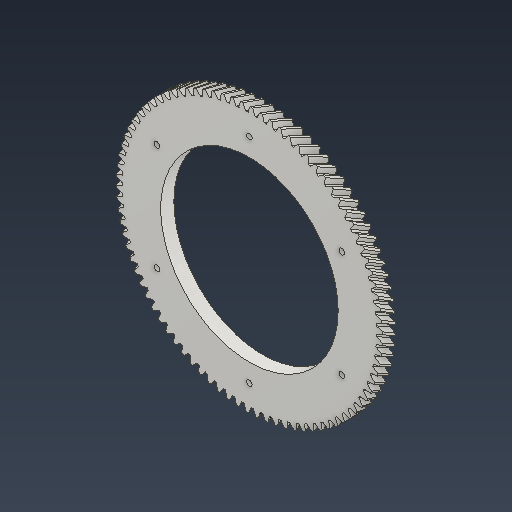
# Autodesk Inventor part: Цилиндрическое зубчатое зацепление2
Saved by Autodesk Inventor 2026 (Build 300175000, 175)
## iProperties
CustomPartVersion: 1
Created: 2025-11-26
Part Number: Цилиндрическое зубчатое зацепление2
Material: Steel
Document SubType Name: Modeling
Designer: Phantom
Categories: <?xml version="1.0" encoding="UTF-16"?> <MemberInstance><Categories><FamilyTemplate><FamilyTemplateParameter ValueType="xs:double" Id="1" ObjectReferenceKey="da_z" ObjectType="kUserParameterObject"/><FamilyTemplateParameter ValueType="xs:double" Id="2" ObjectReferenceKey="da_b" ObjectType="kUserParameterObject"/><FamilyTemplateParameter ValueType="xs:double" Id="3" ObjectReferenceKey="da_beta" ObjectType="kUserParameterObject"/><FamilyTemplateParameter ValueType="xs:double" Id="4" ObjectReferenceKey="da_da" ObjectType="kUserParameterObject"/><FamilyTemplateParameter ValueType="xs:double" Id="5" ObjectReferenceKey="da_aw" ObjectType="kUserParameterObject"/><FamilyTemplateParameter ValueType="xs:string" Id="6" ObjectReferenceKey="EAIAABAAAACIAQAAAAAAAIAAAAAAAAAA" ObjectType="83910656" SubObjectId="SurfaceGeometry"/></FamilyTemplate><ParamToTemplateMap><ParamToTemplate CategoryParameter="//CategoryParameter[@InternalName='046C89C9-8512-4d59-83FE-43B91F4F132A']" TemplateParameter="1"/><ParamToTemplate CategoryParameter="//CategoryParameter[@InternalName='2552DF32-E462-4b46-AEBF-C6C7768E72AC']" TemplateParameter="2"/><ParamToTemplate CategoryParameter="//CategoryParameter[@InternalName='C9EE641D-15FC-4fae-A226-E94C4372FDD7']" TemplateParameter="3"/><ParamToTemplate><ParamToTemplate CategoryParameter="//CategoryParameter[@InternalName='00B6519A-459B-49c7-AD84-2E56D39A5744']" ConstantValue="-0.044335"/></ParamToTemplate><ParamToTemplate><ParamToTemplate CategoryParameter="//CategoryParameter[@InternalName='04B31F0E-C7A6-4894-AA32-9629BEFACF47']" ConstantValue="1.000000"/></ParamToTemplate><ParamToTemplate><ParamToTemplate CategoryParameter="//CategoryParameter[@InternalName='43CBEC2E-7847-49e7-A936-2F7889FCB2D9']" ConstantValue="0.250000"/></ParamToTemplate><ParamToTemplate><ParamToTemplate CategoryParameter="//CategoryParameter[@InternalName='B1EFC894-105D-4ebd-86BF-FA20ED196853']" ConstantValue="0.350000"/></ParamToTemplate><ParamToTemplate><ParamToTemplate CategoryParameter="//CategoryParameter[@InternalName='51175063-3D10-4879-93E8-6246FE8B403D']" ConstantValue="2060000000.000000"/></ParamToTemplate><ParamToTemplate><ParamToTemplate CategoryParameter="//CategoryParameter[@InternalName='A3A52E27-4454-46a9-B0BD-C932399B70AF']" ConstantValue="0.300000"/></ParamToTemplate><ParamToTemplate><ParamToTemplate CategoryParameter="//CategoryParameter[@InternalName='91B76062-C214-41d9-B1B9-14D2AB99603D']" ConstantValue="0.200000"/></ParamToTemplate><ParamToTemplate><ParamToTemplate CategoryParameter="//CategoryParameter[@InternalName='374E806E-8B8A-4dda-A9AA-1039D6500AD2']" ConstantValue="5.000000"/></ParamToTemplate><ParamToTemplate><ParamToTemplate CategoryParameter="//CategoryParameter[@InternalName='2D373A89-B862-43d6-8D0B-0CBF12AB9F6C']" ConstantValue="0.349066"/></ParamToTemplate><ParamToTemplate CategoryParameter="//CategoryParameter[@InternalName='37777632-D6A2-4fac-9D53-DB8ACD95C989']" TemplateParameter="4"/><ParamToTemplate CategoryParameter="//CategoryParameter[@InternalName='FD1017F1-B727-4f7e-9707-0F86F1FF9423']" TemplateParameter="5"/><ParamToTemplate><ParamToTemplate CategoryParameter="//CategoryParameter[@InternalName='9E1B4470-B2D3-4ff1-B813-535BB4CDF51A']" ConstantValue="3520000.000000"/></ParamToTemplate><ParamToTemplate><ParamToTemplate CategoryParameter="//CategoryParameter[@InternalName='F8452263-BFF6-458c-9FB1-07C4B99E95CD']" ConstantValue="11400000.000000"/></ParamToTemplate><ParamToTemplate><ParamToTemplate CategoryParameter="//CategoryParameter[@InternalName='3E3BB259-FD49-497f-8171-6EBC954A3479']" ConstantValue="2.000000"/></ParamToTemplate><ParamToTemplate CategoryParameter="//CategoryParameter[@InternalName='27C3BAF2-7550-4e4b-AE2C-0DB134B7D9B7']" TemplateParameter="6"/></ParamToTemplateMap><Category DisplayName="Gear" InternalName="DC85795E-93AB-48d5-8EEE-5A27447B64BD" Mnemonic="Gear"><CategoryParameter DisplayName="z" InternalName="046C89C9-8512-4d59-83FE-43B91F4F132A" Mnemonic="z"/><CategoryParameter DisplayName="b" InternalName="2552DF32-E462-4b46-AEBF-C6C7768E72AC" Mnemonic="b"/><CategoryParameter DisplayName="||b|" InternalName="C9EE641D-15FC-4fae-A226-E94C4372FDD7" Mnemonic="beta"/><CategoryParameter DisplayName="x" InternalName="00B6519A-459B-49c7-AD84-2E56D39A5744" Mnemonic="x"/><CategoryParameter DisplayName="a*" InternalName="04B31F0E-C7A6-4894-AA32-9629BEFACF47" Mnemonic="a"/><CategoryParameter DisplayName="c*" InternalName="43CBEC2E-7847-49e7-A936-2F7889FCB2D9" Mnemonic="c"/><CategoryParameter DisplayName="r|.f|*" InternalName="B1EFC894-105D-4ebd-86BF-FA20ED196853" Mnemonic="rf"/><CategoryParameter DisplayName="E" InternalName="51175063-3D10-4879-93E8-6246FE8B403D" Mnemonic="E"/><CategoryParameter DisplayName="||m|" InternalName="A3A52E27-4454-46a9-B0BD-C932399B70AF" Mnemonic="mi"/><Category DisplayName="SpurGear" InternalName="26C5A22E-A91E-4dfd-A3B3-23CCAFAE1764" Mnemonic="SpurGear"><CategoryParameter DisplayName="m" InternalName="91B76062-C214-41d9-B1B9-14D2AB99603D" Mnemonic="m"/><CategoryParameter DisplayName="P" InternalName="374E806E-8B8A-4dda-A9AA-1039D6500AD2" Mnemonic="PP"/><CategoryParameter DisplayName="||a|" InternalName="2D373A89-B862-43d6-8D0B-0CBF12AB9F6C" Mnemonic="alpha"/><CategoryParameter DisplayName="d|.a|" InternalName="37777632-D6A2-4fac-9D53-DB8ACD95C989" Mnemonic="da"/><CategoryParameter DisplayName="a|.w|" InternalName="FD1017F1-B727-4f7e-9707-0F86F1FF9423" Mnemonic="aw"/><CategoryParameter DisplayName="||s||.Flim|" InternalName="9E1B4470-B2D3-4ff1-B813-535BB4CDF51A" Mnemonic="sFlim"/><CategoryParameter DisplayName="||s||.Hlim|" InternalName="F8452263-BFF6-458c-9FB1-07C4B99E95CD" Mnemonic="sHlim"/><CategoryParameter DisplayName="тип" InternalName="3E3BB259-FD49-497f-8171-6EBC954A3479" Mnemonic="type"/><CategoryParameter DisplayName="PitchDiameter" InternalName="27C3BAF2-7550-4e4b-AE2C-0DB134B7D9B7" Mnemonic="IDS_PITCHDIAM"/></Category></Category></Categories></MemberInstance>
Density: 1 g/cm^3
Appearance: Steel
d16: 120,000 мм
d17: 0,000 мм
d41: 0,000 мм
d43: 120,000 мм
d46: 120,000 мм
d47: 0,000 мм
d48: 0,000 мм
Author: Phantom
Autodesk Inventor part; units mm, degrees
(part 1 of 2)
sketch "Sketch1" plane through (0, 0, 0) normal (0, 0, 1) x (1, 0, 0)
  circle A0 centre (0, 0) radius 101.2154
  dimension "d0" = 202.4308
  constraints: 1 centre point
  measures "d0" diameter of A0
extrude "Extrusion1" add sketch "Sketch1" along normal blind 10
ref_plane "Work Plane2" through (0, 0, 5) normal (0, 0, 1) x (-0.9983104, -0.0581068, 0)
sketch "Sketch2" plane through (0, 0, 0) normal (0, 0, -1) x (-1, 0, 0)
  circle A0 centre (0, 0) radius 101.2154 projected
  circle A1 centre (0, 0) radius 99.3042
  dimension "d3" = 198.6085
  constraints: 1 centre point, 1 coincident
  measures "d3" diameter of A1
surface extrude "Средний диаметр" sketch "Sketch2" against normal through all shown no curves A1
ref_plane "Work Plane8" through (0, 0, 0) normal (0.9993328, 0.036522, 0) x (0, 0, 1)
ref_plane "Work Plane9" through (0, 0, 0) normal (1, 0, 0) x (0, 1, 0)
spur gear teeth "Цилиндрическое зубчатое зацепление" teeth 86 pitch diameter 198.6085 tip diameter 202.4308 root diameter 193.4312 face width 10 helix angle 30 hand right start plane through (0, 0, 0) normal (0, 0, -1) x (-1, 0, 0)
sketch "Эскиз3" plane through (0, 0, 10) normal (0, 0, 1) x (1, 0, 0)
  circle A0 centre (0, 0) radius 67.5
  dimension "d49" = 135
  constraints: 1 centre point, 1 coincident
  measures "d49" diameter of A0
extrude "Выдавливание2" cut sketch "Эскиз3" against normal through all
sketch "Эскиз4" plane through (0, 0, 10) normal (0, 0, 1) x (1, 0, 0)
  circle A0 centre (0, 0) radius 67.5
  arc A1 (-12.5637, 100.4326) -> (-14.3959, 100.1864) centre (0, 0) ccw
  spline S0 degree 3 poles (-8.4922, 96.342) (-8.7855, 96.3162) (-9.0787, 96.289) (-9.6648, 96.2319) (-9.9577, 96.2021) (-10.2504, 96.1708) knots 0 0 0 0 0.5 0.5 1 1 1 1
  spline S1 degree 3 poles (-1.4371, 96.7049) (-1.7315, 96.7005) (-2.0258, 96.6948) (-2.6145, 96.6807) (-2.9088, 96.6723) (-3.2031, 96.6625) knots 0 0 0 0 0.5 0.5 1 1 1 1
  spline S2 degree 3 poles (0.3447, 101.2148) (-0.0226, 100.4934) (-0.3555, 99.755) (-0.9504, 98.2491) (-1.2121, 97.4826) (-1.4371, 96.7049) knots 0 0 0 0 0.5 0.5 1 1 1 1
  arc A2 (2.1933, 101.1916) -> (0.3447, 101.2148) centre (0, 0) ccw
  spline S3 degree 3 poles (3.8614, 96.6385) (3.656, 97.4215) (3.4136, 98.1944) (2.8566, 99.7147) (2.5423, 100.4612) (2.1933, 101.1916) knots 0 0 0 0 0.5 0.5 1 1 1 1
  spline S4 degree 3 poles (5.6258, 96.5518) (5.3318, 96.5689) (5.0378, 96.5847) (4.4497, 96.6136) (4.1556, 96.6267) (3.8614, 96.6385) knots 0 0 0 0 0.5 0.5 1 1 1 1
  spline S5 degree 3 poles (7.732, 100.9196) (7.313, 100.2269) (6.9271, 99.5148) (6.2238, 98.0564) (5.9069, 97.311) (5.6258, 96.5518) knots 0 0 0 0 0.5 0.5 1 1 1 1
  arc A3 (9.5739, 100.7616) -> (7.732, 100.9196) centre (0, 0) ccw
  spline S6 degree 3 poles (10.9053, 96.0988) (10.7575, 96.8947) (10.5722, 97.6833) (10.1277, 99.2401) (9.8687, 100.0076) (9.5739, 100.7616) knots 0 0 0 0 0.5 0.5 1 1 1 1
  spline S7 degree 3 poles (12.6586, 95.8836) (12.3667, 95.9221) (12.0746, 95.9593) (11.4902, 96.0311) (11.1978, 96.0656) (10.9053, 96.0988) knots 0 0 0 0 0.5 0.5 1 1 1 1
  spline S8 degree 3 poles (15.078, 100.086) (14.6096, 99.4257) (14.1727, 98.7437) (13.3649, 97.3405) (12.9944, 96.6202) (12.6586, 95.8836) knots 0 0 0 0 0.5 0.5 1 1 1 1
  arc A4 (16.9035, 99.7939) -> (15.078, 100.086) centre (0, 0) ccw
  spline S9 degree 3 poles (17.8909, 95.0464) (17.8017, 95.851) (17.6745, 96.651) (17.3448, 98.2361) (17.1425, 99.0205) (16.9035, 99.7939) knots 0 0 0 0 0.5 0.5 1 1 1 1
  spline S10 degree 3 poles (19.6239, 94.7038) (19.3356, 94.7635) (19.047, 94.8219) (18.4694, 94.9361) (18.1803, 94.9919) (17.8909, 95.0464) knots 0 0 0 0 0.5 0.5 1 1 1 1
  spline S11 degree 3 poles (22.3436, 98.7184) (21.8283, 98.0941) (21.3428, 97.4457) (20.4346, 96.1052) (20.0126, 95.4139) (19.6239, 94.7038) knots 0 0 0 0 0.5 0.5 1 1 1 1
  arc A5 (24.1429, 98.2938) -> (22.3436, 98.7184) centre (0, 0) ccw
  spline S12 degree 3 poles (24.7811, 93.4869) (24.7509, 94.2959) (24.6824, 95.103) (24.4693, 96.708) (24.3248, 97.505) (24.1429, 98.2938) knots 0 0 0 0 0.5 0.5 1 1 1 1
  spline S13 degree 3 poles (26.4845, 93.0187) (26.2013, 93.0993) (25.9178, 93.1786) (25.35, 93.3347) (25.0657, 93.4114) (24.7811, 93.4869) knots 0 0 0 0 0.5 0.5 1 1 1 1
  spline S14 degree 3 poles (29.49, 96.824) (28.9304, 96.239) (28.3989, 95.6278) (27.3954, 94.3572) (26.9239, 93.6986) (26.4845, 93.0187) knots 0 0 0 0 0.5 0.5 1 1 1 1
  arc A6 (31.2535, 96.2693) -> (29.49, 96.824) centre (0, 0) ccw
  spline S15 degree 3 poles (31.5391, 91.4286) (31.568, 92.2376) (31.5586, 93.0476) (31.4632, 94.6638) (31.3773, 95.4693) (31.2535, 96.2693) knots 0 0 0 0 0.5 0.5 1 1 1 1
  spline S16 degree 3 poles (33.2037, 90.8373) (32.9272, 90.9384) (32.6502, 91.0382) (32.0953, 91.2353) (31.8175, 91.3326) (31.5391, 91.4286) knots 0 0 0 0 0.5 0.5 1 1 1 1
  spline S17 degree 3 poles (36.479, 94.4131) (35.8783, 93.8705) (35.3035, 93.2997) (34.2099, 92.1058) (33.6917, 91.4833) (33.2037, 90.8373) knots 0 0 0 0 0.5 0.5 1 1 1 1
  arc A7 (38.1973, 93.7311) -> (36.479, 94.4131) centre (0, 0) ccw
  spline S18 degree 3 poles (38.1289, 88.8825) (38.2167, 89.6872) (38.2664, 90.4957) (38.2893, 92.1146) (38.2624, 92.9242) (38.1973, 93.7311) knots 0 0 0 0 0.5 0.5 1 1 1 1
  spline S19 degree 3 poles (39.7459, 88.1713) (39.4774, 88.2922) (39.2085, 88.412) (38.6695, 88.6491) (38.3994, 88.7664) (38.1289, 88.8825) knots 0 0 0 0 0.5 0.5 1 1 1 1
  spline S20 degree 3 poles (43.2734, 91.4984) (42.6347, 91.0011) (42.0198, 90.4738) (40.8419, 89.3629) (40.2796, 88.7799) (39.7459, 88.1713) knots 0 0 0 0 0.5 0.5 1 1 1 1
  arc A8 (44.9373, 90.6928) -> (43.2734, 91.4984) centre (0, 0) ccw
  spline S21 degree 3 poles (44.5151, 85.8621) (44.6615, 86.6583) (44.7701, 87.461) (44.9111, 89.074) (44.9434, 89.8833) (44.9373, 90.6928) knots 0 0 0 0 0.5 0.5 1 1 1 1
  spline S22 degree 3 poles (46.0759, 85.0348) (45.817, 85.175) (45.5575, 85.3141) (45.0373, 85.5899) (44.7765, 85.7266) (44.5151, 85.8621) knots 0 0 0 0 0.5 0.5 1 1 1 1
  spline S23 degree 3 poles (49.8369, 88.0956) (49.1636, 87.6462) (48.5119, 87.1652) (47.2561, 86.1432) (46.6527, 85.6028) (46.0759, 85.0348) knots 0 0 0 0 0.5 0.5 1 1 1 1
  arc A9 (51.4376, 87.1707) -> (49.8369, 88.0956) centre (0, 0) ccw
  spline S24 degree 3 poles (50.6639, 82.3837) (50.868, 83.1671) (51.0349, 83.9597) (51.2933, 85.558) (51.3845, 86.3629) (51.4376, 87.1707) knots 0 0 0 0 0.5 0.5 1 1 1 1
  spline S25 degree 3 poles (52.1601, 81.4446) (51.9122, 81.6034) (51.6635, 81.761) (51.1648, 82.0741) (50.9147, 82.2294) (50.6639, 82.3837) knots 0 0 0 0 0.5 0.5 1 1 1 1
  spline S26 degree 3 poles (56.1346, 84.2227) (55.4302, 83.8237) (54.7451, 83.3916) (53.4181, 82.464) (52.7769, 81.969) (52.1601, 81.4446) knots 0 0 0 0 0.5 0.5 1 1 1 1
  arc A10 (57.6634, 83.1834) -> (56.1346, 84.2227) centre (0, 0) ccw
  spline S27 degree 3 poles (56.5424, 78.4657) (56.8031, 79.2321) (57.0275, 80.0104) (57.4018, 81.5856) (57.5515, 82.3817) (57.6634, 83.1834) knots 0 0 0 0 0.5 0.5 1 1 1 1
  spline S28 degree 3 poles (57.9661, 77.4199) (57.7304, 77.5963) (57.4939, 77.7717) (57.0193, 78.1203) (56.7813, 78.2935) (56.5424, 78.4657) knots 0 0 0 0 0.5 0.5 1 1 1 1
  spline S29 degree 3 poles (62.1327, 79.9005) (61.401, 79.5539) (60.6862, 79.173) (59.295, 78.3447) (58.6194, 77.8979) (57.9661, 77.4199) knots 0 0 0 0 0.5 0.5 1 1 1 1
  arc A11 (63.5816, 78.7524) -> (62.1327, 79.9005) centre (0, 0) ccw
  spline S30 degree 3 poles (62.1192, 74.129) (62.4352, 74.8743) (62.7157, 75.6342) (63.204, 77.1779) (63.4115, 77.9609) (63.5816, 78.7524) knots 0 0 0 0 0.5 0.5 1 1 1 1
  spline S31 degree 3 poles (63.4627, 72.9821) (63.2405, 73.1753) (63.0175, 73.3675) (62.5696, 73.7498) (62.3448, 73.9399) (62.1192, 74.129) knots 0 0 0 0 0.5 0.5 1 1 1 1
  spline S32 degree 3 poles (67.7993, 75.1519) (67.0443, 74.8597) (66.3036, 74.5319) (64.8556, 73.8074) (64.1492, 73.4111) (63.4627, 72.9821) knots 0 0 0 0 0.5 0.5 1 1 1 1
  arc A12 (69.1606, 73.9011) -> (67.7993, 75.1519) centre (0, 0) ccw
  spline S33 degree 3 poles (67.3645, 69.3969) (67.7341, 70.1171) (68.0693, 70.8545) (68.669, 72.3584) (68.9331, 73.1242) (69.1606, 73.9011) knots 0 0 0 0 0.5 0.5 1 1 1 1
  spline S34 degree 3 poles (68.6208, 68.1549) (68.4133, 68.3638) (68.2049, 68.5718) (67.7861, 68.9857) (67.5758, 69.1918) (67.3645, 69.3969) knots 0 0 0 0 0.5 0.5 1 1 1 1
  spline S35 degree 3 poles (73.1041, 70.0024) (72.3299, 69.7661) (71.5672, 69.4933) (70.0702, 68.8764) (69.3368, 68.5327) (68.6208, 68.1549) knots 0 0 0 0 0.5 0.5 1 1 1 1
  arc A13 (74.3705, 68.6556) -> (73.1041, 70.0024) centre (0, 0) ccw
  spline S36 degree 3 poles (72.2505, 64.2944) (72.6716, 64.9858) (73.0598, 65.6967) (73.7677, 67.1529) (74.0869, 67.8973) (74.3705, 68.6556) knots 0 0 0 0 0.5 0.5 1 1 1 1
  spline S37 degree 3 poles (73.4127, 62.9641) (73.221, 63.1876) (73.0283, 63.4102) (72.6409, 63.8536) (72.4462, 64.0745) (72.2505, 64.2944) knots 0 0 0 0 0.5 0.5 1 1 1 1
  spline S38 degree 3 poles (78.019, 64.4794) (77.2295, 64.3002) (76.449, 64.0838) (74.911, 63.5778) (74.1544, 63.2886) (73.4127, 62.9641) knots 0 0 0 0 0.5 0.5 1 1 1 1
  arc A14 (79.1836, 63.0437) -> (78.019, 64.4794) centre (0, 0) ccw
  spline S39 degree 3 poles (76.7509, 58.849) (77.2214, 59.5078) (77.6604, 60.1884) (78.4727, 61.589) (78.8455, 62.3082) (79.1836, 63.0437) knots 0 0 0 0 0.5 0.5 1 1 1 1
  spline S40 degree 3 poles (77.8129, 57.4374) (77.6381, 57.6742) (77.4622, 57.9103) (77.1081, 58.3809) (76.9301, 58.6153) (76.7509, 58.849) knots 0 0 0 0 0.5 0.5 1 1 1 1
  spline S41 degree 3 poles (82.5175, 58.6124) (81.7171, 58.4913) (80.9228, 58.3324) (79.352, 57.9401) (78.5763, 57.7069) (77.8129, 57.4374) knots 0 0 0 0 0.5 0.5 1 1 1 1
  arc A15 (83.5743, 57.0955) -> (82.5175, 58.6124) centre (0, 0) ccw
  spline S42 degree 3 poles (80.8419, 53.0895) (81.3592, 53.7122) (81.8467, 54.359) (82.7591, 55.6966) (83.1833, 56.3866) (83.5743, 57.0955) knots 0 0 0 0 0.5 0.5 1 1 1 1
  spline S43 degree 3 poles (81.798, 51.6042) (81.6409, 51.8532) (81.4827, 52.1015) (81.164, 52.5966) (81.0035, 52.8434) (80.8419, 53.0895) knots 0 0 0 0 0.5 0.5 1 1 1 1
  spline S44 degree 3 poles (86.5758, 52.4326) (85.7687, 52.3703) (84.9649, 52.2698) (83.3697, 51.9932) (82.579, 51.8172) (81.798, 51.6042) knots 0 0 0 0 0.5 0.5 1 1 1 1
  arc A16 (87.519, 50.8427) -> (86.5758, 52.4326) centre (0, 0) ccw
  spline S45 degree 3 poles (84.5015, 47.0468) (85.0629, 47.6301) (85.5964, 48.2396) (86.6039, 49.507) (87.0774, 50.1642) (87.519, 50.8427) knots 0 0 0 0 0.5 0.5 1 1 1 1
  spline S46 degree 3 poles (85.3467, 45.4956) (85.2082, 45.7554) (85.0685, 46.0146) (84.7867, 46.5317) (84.6447, 46.7896) (84.5015, 47.0468) knots 0 0 0 0 0.5 0.5 1 1 1 1
  spline S47 degree 3 poles (90.1722, 45.9731) (89.3627, 45.9699) (88.5537, 45.9283) (86.9425, 45.7689) (86.1411, 45.6511) (85.3467, 45.4956) knots 0 0 0 0 0.5 0.5 1 1 1 1
  arc A17 (90.9968, 44.3185) -> (90.1722, 45.9731) centre (0, 0) ccw
  spline S48 degree 3 poles (87.7103, 40.7531) (88.3127, 41.2938) (88.8893, 41.8628) (89.9866, 43.0532) (90.5068, 43.6741) (90.9968, 44.3185) knots 0 0 0 0 0.5 0.5 1 1 1 1
  spline S49 degree 3 poles (88.4399, 39.1443) (88.3208, 39.4136) (88.2004, 39.6823) (87.9572, 40.2185) (87.8343, 40.4861) (87.7103, 40.7531) knots 0 0 0 0 0.5 0.5 1 1 1 1
  spline S50 degree 3 poles (93.2875, 39.2683) (92.4799, 39.3242) (91.6701, 39.3418) (90.0515, 39.3004) (89.2436, 39.2414) (88.4399, 39.1443) knots 0 0 0 0 0.5 0.5 1 1 1 1
  arc A18 (93.9891, 37.558) -> (93.2875, 39.2683) centre (0, 0) ccw
  spline S51 degree 3 poles (90.4511, 34.2419) (91.0914, 34.7372) (91.7079, 35.2626) (92.8893, 36.3698) (93.4534, 36.951) (93.9891, 37.558) knots 0 0 0 0 0.5 0.5 1 1 1 1
  spline S52 degree 3 poles (91.0614, 32.5842) (90.9622, 32.8614) (90.8617, 33.1382) (90.6583, 33.6908) (90.5553, 33.9666) (90.4511, 34.2419) knots 0 0 0 0 0.5 0.5 1 1 1 1
  spline S53 degree 3 poles (95.905, 32.354) (95.1036, 32.4687) (94.2973, 32.5454) (92.68, 32.6222) (91.87, 32.6224) (91.0614, 32.5842) knots 0 0 0 0 0.5 0.5 1 1 1 1
  arc A19 (96.4799, 30.597) -> (95.905, 32.354) centre (0, 0) ccw
  spline S54 degree 3 poles (92.7093, 27.5481) (93.384, 27.9953) (94.0373, 28.4743) (95.2963, 29.4923) (95.9013, 30.0308) (96.4799, 30.597) knots 0 0 0 0 0.5 0.5 1 1 1 1
  spline S55 degree 3 poles (93.1969, 25.8502) (93.1182, 26.1339) (93.0383, 26.4173) (92.8757, 26.9833) (92.7931, 27.2659) (92.7093, 27.5481) knots 0 0 0 0 0.5 0.5 1 1 1 1
  spline S56 degree 3 poles (98.0109, 25.2671) (97.22, 25.44) (96.4214, 25.5753) (94.814, 25.77) (94.0062, 25.8293) (93.1969, 25.8502) knots 0 0 0 0 0.5 0.5 1 1 1 1
  arc A20 (98.456, 23.4728) -> (98.0109, 25.2671) centre (0, 0) ccw
  spline S57 degree 3 poles (94.4728, 20.7072) (95.1784, 21.104) (95.8649, 21.534) (97.1949, 22.4574) (97.8376, 22.9503) (98.456, 23.4728) knots 0 0 0 0 0.5 0.5 1 1 1 1
  spline S58 degree 3 poles (94.8353, 18.9783) (94.7775, 19.267) (94.7184, 19.5555) (94.5976, 20.1318) (94.5359, 20.4197) (94.4728, 20.7072) knots 0 0 0 0 0.5 0.5 1 1 1 1
  spline S59 degree 3 poles (99.5938, 18.0454) (98.8176, 18.2755) (98.031, 18.4687) (96.4422, 18.7803) (95.6408, 18.8983) (94.8353, 18.9783) knots 0 0 0 0 0.5 0.5 1 1 1 1
  arc A21 (99.9067, 16.2234) -> (99.5938, 18.0454) centre (0, 0) ccw
  spline S60 degree 3 poles (95.7323, 13.7559) (96.465, 14.1002) (97.181, 14.4789) (98.5749, 15.3027) (99.2519, 15.7474) (99.9067, 16.2234) knots 0 0 0 0 0.5 0.5 1 1 1 1
  spline S61 degree 3 poles (95.9676, 12.0052) (95.931, 12.2973) (95.8932, 12.5893) (95.8147, 13.1729) (95.7742, 13.4645) (95.7323, 13.7559) knots 0 0 0 0 0.5 0.5 1 1 1 1
  spline S62 degree 3 poles (100.6453, 10.7273) (99.888, 11.0135) (99.1176, 11.2637) (97.5558, 11.6903) (96.7652, 11.8666) (95.9676, 12.0052) knots 0 0 0 0 0.5 0.5 1 1 1 1
  arc A22 (100.8245, 8.8874) -> (100.6453, 10.7273) centre (0, 0) ccw
  spline S63 degree 3 poles (96.4811, 6.7312) (97.2369, 7.0211) (97.9787, 7.3465) (99.4289, 8.0664) (100.1366, 8.4605) (100.8245, 8.8874) knots 0 0 0 0 0.5 0.5 1 1 1 1
  spline S64 degree 3 poles (96.5879, 4.968) (96.5728, 5.262) (96.5563, 5.556) (96.5207, 6.1437) (96.5015, 6.4375) (96.4811, 6.7312) knots 0 0 0 0 0.5 0.5 1 1 1 1
  spline S65 degree 3 poles (101.1599, 3.3521) (100.4255, 3.6928) (99.6754, 3.9985) (98.1489, 4.538) (97.3732, 4.7715) (96.5879, 4.968) knots 0 0 0 0 0.5 0.5 1 1 1 1
  arc A23 (101.2042, 1.5039) -> (101.1599, 3.3521) centre (0, 0) ccw
  spline S66 degree 3 poles (96.715, -0.3294) (97.49, -0.0955) (98.2536, 0.1749) (99.7525, 0.7871) (100.487, 1.1284) (101.2042, 1.5039) knots 0 0 0 0 0.5 0.5 1 1 1 1
  spline S67 degree 3 poles (96.6929, -2.0957) (96.6992, -1.8014) (96.7043, -1.507) (96.7117, -0.9182) (96.714, -0.6238) (96.715, -0.3294) knots 0 0 0 0 0.5 0.5 1 1 1 1
  spline S68 degree 3 poles (101.1347, -4.0411) (100.4271, -3.6477) (99.7014, -3.288) (98.2183, -2.6385) (97.4618, -2.349) (96.6929, -2.0957) knots 0 0 0 0 0.5 0.5 1 1 1 1
  arc A24 (101.044, -5.8875) -> (101.1347, -4.0411) centre (0, 0) ccw
  spline S69 degree 3 poles (96.433, -7.3883) (97.223, -7.2116) (98.0042, -6.9976) (99.5438, -6.4965) (100.3013, -6.2097) (101.044, -5.8875) knots 0 0 0 0 0.5 0.5 1 1 1 1
  spline S70 degree 3 poles (96.2819, -9.1483) (96.3098, -8.8552) (96.3363, -8.562) (96.3866, -7.9753) (96.4105, -7.6818) (96.433, -7.3883) knots 0 0 0 0 0.5 0.5 1 1 1 1
  spline S71 degree 3 poles (100.5699, -11.4126) (99.893, -10.9687) (99.1954, -10.557) (97.7637, -9.8009) (97.0303, -9.457) (96.2819, -9.1483) knots 0 0 0 0 0.5 0.5 1 1 1 1
  arc A25 (100.3447, -13.2475) -> (100.5699, -11.4126) centre (0, 0) ccw
  spline S72 degree 3 poles (95.6364, -14.4077) (96.4372, -14.2892) (97.232, -14.1328) (98.804, -13.7454) (99.5805, -13.5146) (100.3447, -13.2475) knots 0 0 0 0 0.5 0.5 1 1 1 1
  spline S73 degree 3 poles (95.3573, -16.152) (95.4065, -15.8617) (95.4543, -15.5712) (95.5474, -14.9898) (95.5925, -14.6988) (95.6364, -14.4077) knots 0 0 0 0 0.5 0.5 1 1 1 1
  spline S74 degree 3 poles (99.4685, -18.7233) (98.8258, -18.2311) (98.1602, -17.7696) (96.7874, -16.9111) (96.0812, -16.5145) (95.3573, -16.152) knots 0 0 0 0 0.5 0.5 1 1 1 1
  arc A26 (99.11, -20.5369) -> (99.4685, -18.7233) centre (0, 0) ccw
  spline S75 degree 3 poles (94.3296, -21.3503) (95.1369, -21.2905) (95.941, -21.1926) (97.5371, -20.921) (98.3283, -20.7475) (99.11, -20.5369) knots 0 0 0 0 0.5 0.5 1 1 1 1
  spline S76 degree 3 poles (93.9239, -23.0696) (93.9941, -22.7836) (94.063, -22.4974) (94.1983, -21.9243) (94.2646, -21.6374) (94.3296, -21.3503) knots 0 0 0 0 0.5 0.5 1 1 1 1
  spline S77 degree 3 poles (97.8365, -25.9341) (97.2314, -25.3963) (96.6012, -24.8874) (95.2948, -23.931) (94.6194, -23.4839) (93.9239, -23.0696) knots 0 0 0 0 0.5 0.5 1 1 1 1
  arc A27 (97.3465, -27.7167) -> (97.8365, -25.9341) centre (0, 0) ccw
  spline S78 degree 3 poles (92.5195, -28.1789) (93.329, -28.1783) (94.1381, -28.1393) (95.7498, -27.9849) (96.5515, -27.8697) (97.3465, -27.7167) knots 0 0 0 0 0.5 0.5 1 1 1 1
  spline S79 degree 3 poles (91.9894, -29.864) (92.0803, -29.584) (92.1699, -29.3035) (92.3466, -28.7418) (92.4337, -28.4606) (92.5195, -28.1789) knots 0 0 0 0 0.5 0.5 1 1 1 1
  spline S80 degree 3 poles (95.6824, -33.0065) (95.1182, -32.426) (94.5268, -31.8725) (93.2937, -30.8232) (92.6527, -30.328) (91.9894, -29.864) knots 0 0 0 0 0.5 0.5 1 1 1 1
  arc A28 (95.0636, -34.7486) -> (95.6824, -33.0065) centre (0, 0) ccw
  spline S81 degree 3 poles (90.2157, -34.8573) (91.0231, -34.9157) (91.8329, -34.9358) (93.4516, -34.8995) (94.2596, -34.8431) (95.0636, -34.7486) knots 0 0 0 0 0.5 0.5 1 1 1 1
  spline S82 degree 3 poles (89.564, -36.4991) (89.6751, -36.2265) (89.785, -35.9533) (90.0022, -35.406) (90.1096, -35.1319) (90.2157, -34.8573) knots 0 0 0 0 0.5 0.5 1 1 1 1
  spline S83 degree 3 poles (93.0178, -39.9028) (92.4975, -39.2827) (91.9481, -38.6875) (90.7949, -37.551) (90.1917, -37.0104) (89.564, -36.4991) knots 0 0 0 0 0.5 0.5 1 1 1 1
  arc A29 (92.2735, -41.5951) -> (93.0178, -39.9028) centre (0, 0) ccw
  spline S84 degree 3 poles (87.4306, -41.3496) (88.2316, -41.4668) (89.0378, -41.546) (90.6548, -41.628) (91.4648, -41.6307) (92.2735, -41.5951) knots 0 0 0 0 0.5 0.5 1 1 1 1
  spline S85 degree 3 poles (86.6608, -42.9395) (86.7915, -42.6757) (86.9211, -42.4113) (87.1777, -41.8813) (87.3048, -41.6157) (87.4306, -41.3496) knots 0 0 0 0 0.5 0.5 1 1 1 1
  spline S86 degree 3 poles (89.857, -46.5863) (89.3833, -45.9298) (88.8788, -45.296) (87.8117, -44.0784) (87.2496, -43.4952) (86.6608, -42.9395) knots 0 0 0 0 0.5 0.5 1 1 1 1
  arc A30 (88.9911, -48.2196) -> (89.857, -46.5863) centre (0, 0) ccw
  spline S87 degree 3 poles (84.1791, -47.6213) (84.9694, -47.7967) (85.7676, -47.9345) (87.3743, -48.1343) (88.1819, -48.1961) (88.9911, -48.2196) knots 0 0 0 0 0.5 0.5 1 1 1 1
  spline S88 degree 3 poles (83.2953, -49.1508) (83.4449, -48.8972) (83.5934, -48.643) (83.888, -48.1332) (84.0341, -47.8776) (84.1791, -47.6213) knots 0 0 0 0 0.5 0.5 1 1 1 1
  spline S89 degree 3 poles (86.2167, -53.0211) (85.7922, -52.3318) (85.3353, -51.6629) (84.3599, -50.3707) (83.8419, -49.748) (83.2953, -49.1508) knots 0 0 0 0 0.5 0.5 1 1 1 1
  arc A31 (85.2339, -54.5869) -> (86.2167, -53.0211) centre (0, 0) ccw
  spline S90 degree 3 poles (80.4784, -53.6389) (81.2538, -53.8715) (82.0398, -54.0673) (83.6276, -54.3838) (84.4286, -54.5044) (85.2339, -54.5869) knots 0 0 0 0 0.5 0.5 1 1 1 1
  spline S91 degree 3 poles (79.4853, -55.0999) (79.653, -54.8579) (79.8196, -54.6152) (80.1507, -54.1282) (80.3151, -53.8839) (80.4784, -53.6389) knots 0 0 0 0 0.5 0.5 1 1 1 1
  spline S92 degree 3 poles (82.1164, -59.1731) (81.7433, -58.4546) (81.3365, -57.7542) (80.458, -56.3942) (79.9868, -55.7353) (79.4853, -55.0999) knots 0 0 0 0 0.5 0.5 1 1 1 1
  arc A32 (81.0219, -60.663) -> (82.1164, -59.1731) centre (0, 0) ccw
  spline S93 degree 3 poles (76.3483, -59.3704) (77.1047, -59.6589) (77.8743, -59.9116) (79.4348, -60.3431) (80.2248, -60.5219) (81.0219, -60.663) knots 0 0 0 0 0.5 0.5 1 1 1 1
  spline S94 degree 3 poles (75.2512, -60.7549) (75.4361, -60.5258) (75.6201, -60.2959) (75.9857, -59.8344) (76.1675, -59.6028) (76.3483, -59.3704) knots 0 0 0 0 0.5 0.5 1 1 1 1
  spline S95 degree 3 poles (77.578, -65.0093) (77.2584, -64.2656) (76.9038, -63.5373) (76.1269, -62.1168) (75.705, -61.4253) (75.2512, -60.7549) knots 0 0 0 0 0.5 0.5 1 1 1 1
  arc A33 (76.3777, -66.4154) -> (77.578, -65.0093) centre (0, 0) ccw
  spline S96 degree 3 poles (71.8108, -64.7851) (72.5441, -65.1281) (73.2932, -65.4362) (74.8181, -65.9805) (75.593, -66.2165) (76.3777, -66.4154) knots 0 0 0 0 0.5 0.5 1 1 1 1
  spline S97 degree 3 poles (70.6156, -66.0858) (70.8168, -65.8709) (71.017, -65.655) (71.4154, -65.2214) (71.6136, -65.0037) (71.8108, -64.7851) knots 0 0 0 0 0.5 0.5 1 1 1 1
  spline S98 degree 3 poles (72.6256, -70.4987) (72.3612, -69.7336) (72.0607, -68.9814) (71.3895, -67.508) (71.0193, -66.7875) (70.6156, -66.0858) knots 0 0 0 0 0.5 0.5 1 1 1 1
  arc A34 (71.3259, -71.8134) -> (72.6256, -70.4987) centre (0, 0) ccw
  spline S99 degree 3 poles (66.8903, -69.8541) (67.5966, -70.2497) (68.3212, -70.6117) (69.8022, -71.2659) (70.5578, -71.5578) (71.3259, -71.8134) knots 0 0 0 0 0.5 0.5 1 1 1 1
  spline S100 degree 3 poles (65.6033, -71.0641) (65.8196, -70.8644) (66.035, -70.6637) (66.464, -70.2604) (66.6776, -70.0577) (66.8903, -69.8541) knots 0 0 0 0 0.5 0.5 1 1 1 1
  spline S101 degree 3 poles (67.2858, -75.612) (67.0779, -74.8296) (66.8331, -74.0575) (66.2713, -72.539) (65.9547, -71.7934) (65.6033, -71.0641) knots 0 0 0 0 0.5 0.5 1 1 1 1
  arc A35 (65.8936, -76.8283) -> (67.2858, -75.612) centre (0, 0) ccw
  spline S102 degree 3 poles (61.6128, -74.5504) (62.2883, -74.9965) (62.9846, -75.4104) (64.4139, -76.171) (65.1462, -76.5173) (65.8936, -76.8283) knots 0 0 0 0 0.5 0.5 1 1 1 1
  spline S103 degree 3 poles (60.2409, -75.6633) (60.4713, -75.4799) (60.7008, -75.2955) (61.1581, -74.9245) (61.3859, -74.738) (61.6128, -74.5504) knots 0 0 0 0 0.5 0.5 1 1 1 1
  spline S104 degree 3 poles (61.587, -80.3218) (61.4368, -79.5264) (61.249, -78.7384) (60.7995, -77.183) (60.5381, -76.4163) (60.2409, -75.6633) knots 0 0 0 0 0.5 0.5 1 1 1 1
  arc A36 (60.1097, -81.4333) -> (61.587, -80.3218) centre (0, 0) ccw
  spline S105 degree 3 poles (56.0066, -78.849) (56.6478, -79.3432) (57.312, -79.8068) (58.682, -80.6697) (59.387, -81.0685) (60.1097, -81.4333) knots 0 0 0 0 0.5 0.5 1 1 1 1
  spline S106 degree 3 poles (54.5572, -79.8587) (54.8003, -79.6927) (55.0426, -79.5255) (55.5258, -79.1889) (55.7666, -79.0195) (56.0066, -78.849) knots 0 0 0 0 0.5 0.5 1 1 1 1
  spline S107 degree 3 poles (55.5596, -84.6031) (55.4678, -83.7988) (55.338, -82.9993) (55.0033, -81.4151) (54.7986, -80.6314) (54.5572, -79.8587) knots 0 0 0 0 0.5 0.5 1 1 1 1
  arc A37 (54.0051, -85.6038) -> (55.5596, -84.6031) centre (0, 0) ccw
  spline S108 degree 3 poles (50.1016, -82.7269) (50.705, -83.2666) (51.3336, -83.7774) (52.6369, -84.738) (53.311, -85.1872) (54.0051, -85.6038) knots 0 0 0 0 0.5 0.5 1 1 1 1
  spline S109 degree 3 poles (48.5823, -83.6281) (48.8369, -83.4802) (49.0908, -83.3312) (49.5972, -83.0308) (49.8497, -82.8794) (50.1016, -82.7269) knots 0 0 0 0 0.5 0.5 1 1 1 1
  spline S110 degree 3 poles (49.2357, -88.433) (49.2029, -87.6241) (49.1319, -86.8173) (48.9137, -85.2129) (48.7667, -84.4164) (48.5823, -83.6281) knots 0 0 0 0 0.5 0.5 1 1 1 1
  arc A38 (47.6124, -89.3175) -> (49.2357, -88.433) centre (0, 0) ccw
  spline S111 degree 3 poles (43.9293, -86.1634) (44.4916, -86.7457) (45.0812, -87.3011) (46.311, -88.3542) (46.9505, -88.8514) (47.6124, -89.3175) knots 0 0 0 0 0.5 0.5 1 1 1 1
  spline S112 degree 3 poles (42.3482, -86.9513) (42.6129, -86.8224) (42.877, -86.6923) (43.4041, -86.4296) (43.667, -86.2971) (43.9293, -86.1634) knots 0 0 0 0 0.5 0.5 1 1 1 1
  spline S113 degree 3 poles (42.6492, -91.7911) (42.6755, -90.982) (42.6635, -90.1721) (42.563, -88.5561) (42.4746, -87.7509) (42.3482, -86.9513) knots 0 0 0 0 0.5 0.5 1 1 1 1
  arc A39 (40.9656, -92.5547) -> (42.6492, -91.7911) centre (0, 0) ccw
  spline S114 degree 3 poles (37.5225, -89.1401) (38.0409, -89.7619) (38.5884, -90.3589) (39.738, -91.499) (40.3395, -92.0415) (40.9656, -92.5547) knots 0 0 0 0 0.5 0.5 1 1 1 1
  spline S115 degree 3 poles (35.8882, -89.8106) (36.1616, -89.7013) (36.4345, -89.5908) (36.9793, -89.3673) (37.2512, -89.2543) (37.5225, -89.1401) knots 0 0 0 0 0.5 0.5 1 1 1 1
  spline S116 degree 3 poles (35.8351, -94.6594) (35.9204, -93.8544) (35.9676, -93.0457) (35.9853, -91.4267) (35.9559, -90.6173) (35.8882, -89.8106) knots 0 0 0 0 0.5 0.5 1 1 1 1
  arc A40 (34.1002, -95.2981) -> (35.8351, -94.6594) centre (0, 0) ccw
  spline S117 degree 3 poles (30.9156, -91.6413) (31.3872, -92.2993) (31.8897, -92.9346) (32.953, -94.1556) (33.5133, -94.7406) (34.1002, -95.2981) knots 0 0 0 0 0.5 0.5 1 1 1 1
  spline S118 degree 3 poles (29.2367, -92.1907) (29.5174, -92.1016) (29.7976, -92.0114) (30.3573, -91.8282) (30.6367, -91.7354) (30.9156, -91.6413) knots 0 0 0 0 0.5 0.5 1 1 1 1
  spline S119 degree 3 poles (28.8298, -97.0227) (28.9736, -96.226) (29.0797, -95.423) (29.2156, -93.8096) (29.2453, -93.0002) (29.2367, -92.1907) knots 0 0 0 0 0.5 0.5 1 1 1 1
  arc A41 (27.053, -97.533) -> (28.8298, -97.0227) centre (0, 0) ccw
  spline S120 degree 3 poles (24.1438, -93.6535) (24.5661, -94.3442) (25.0208, -95.0145) (25.9922, -96.3098) (26.5082, -96.9342) (27.053, -97.533) knots 0 0 0 0 0.5 0.5 1 1 1 1
  spline S121 degree 3 poles (22.4293, -94.0789) (22.7156, -94.0106) (23.0017, -93.941) (23.5732, -93.7992) (23.8587, -93.727) (24.1438, -93.6535) knots 0 0 0 0 0.5 0.5 1 1 1 1
  spline S122 degree 3 poles (21.6707, -98.8683) (21.8723, -98.0842) (22.0367, -97.2911) (22.29, -95.6919) (22.3787, -94.8868) (22.4293, -94.0789) knots 0 0 0 0 0.5 0.5 1 1 1 1
  arc A42 (19.8613, -99.2476) -> (21.6707, -98.8683) centre (0, 0) ccw
  spline S123 degree 3 poles (17.2431, -95.1661) (17.6139, -95.8857) (18.0185, -96.5874) (18.8927, -97.9502) (19.3618, -98.6105) (19.8613, -99.2476) knots 0 0 0 0 0.5 0.5 1 1 1 1
  spline S124 degree 3 poles (15.5021, -95.4651) (15.7927, -95.4179) (16.0831, -95.3694) (16.6635, -95.2697) (16.9534, -95.2185) (17.2431, -95.1661) knots 0 0 0 0 0.5 0.5 1 1 1 1
  spline S125 degree 3 poles (14.3959, -100.1864) (14.6543, -99.4192) (14.8761, -98.6401) (15.2455, -97.0637) (15.3927, -96.2672) (15.5021, -95.4651) knots 0 0 0 0 0.5 0.5 1 1 1 1
  arc A43 (12.5637, -100.4326) -> (14.3959, -100.1864) centre (0, 0) ccw
  spline S126 degree 3 poles (10.2504, -96.1708) (10.5677, -96.9156) (10.92, -97.645) (11.6924, -99.068) (12.112, -99.7608) (12.5637, -100.4326) knots 0 0 0 0 0.5 0.5 1 1 1 1
  spline S127 degree 3 poles (8.4922, -96.342) (8.7855, -96.3162) (9.0787, -96.289) (9.6648, -96.2319) (9.9577, -96.2021) (10.2504, -96.1708) knots 0 0 0 0 0.5 0.5 1 1 1 1
  spline S128 degree 3 poles (7.0444, -100.97) (7.358, -100.2236) (7.6362, -99.4629) (8.1196, -97.9176) (8.3246, -97.134) (8.4922, -96.342) knots 0 0 0 0 0.5 0.5 1 1 1 1
  arc A44 (5.1991, -101.0818) -> (7.0444, -100.97) centre (0, 0) ccw
  spline S129 degree 3 poles (3.2031, -96.6625) (3.4651, -97.4285) (3.7632, -98.1816) (4.4297, -99.6572) (4.7977, -100.3788) (5.1991, -101.0818) knots 0 0 0 0 0.5 0.5 1 1 1 1
  spline S130 degree 3 poles (1.4371, -96.7049) (1.7315, -96.7005) (2.0258, -96.6948) (2.6145, -96.6807) (2.9088, -96.6723) (3.2031, -96.6625) knots 0 0 0 0 0.5 0.5 1 1 1 1
  spline S131 degree 3 poles (-0.3447, -101.2148) (0.0226, -100.4934) (0.3555, -99.755) (0.9504, -98.2491) (1.2121, -97.4826) (1.4371, -96.7049) knots 0 0 0 0 0.5 0.5 1 1 1 1
  arc A45 (-2.1933, -101.1916) -> (-0.3447, -101.2148) centre (0, 0) ccw
  spline S132 degree 3 poles (-3.8614, -96.6385) (-3.656, -97.4215) (-3.4136, -98.1944) (-2.8566, -99.7147) (-2.5423, -100.4612) (-2.1933, -101.1916) knots 0 0 0 0 0.5 0.5 1 1 1 1
  spline S133 degree 3 poles (-5.6258, -96.5518) (-5.3318, -96.5689) (-5.0378, -96.5847) (-4.4497, -96.6136) (-4.1556, -96.6267) (-3.8614, -96.6385) knots 0 0 0 0 0.5 0.5 1 1 1 1
  spline S134 degree 3 poles (-7.732, -100.9196) (-7.313, -100.2269) (-6.9271, -99.5148) (-6.2238, -98.0564) (-5.9069, -97.311) (-5.6258, -96.5518) knots 0 0 0 0 0.5 0.5 1 1 1 1
  arc A46 (-9.5739, -100.7616) -> (-7.732, -100.9196) centre (0, 0) ccw
  spline S135 degree 3 poles (-10.9053, -96.0988) (-10.7575, -96.8947) (-10.5722, -97.6833) (-10.1277, -99.2401) (-9.8687, -100.0076) (-9.5739, -100.7616) knots 0 0 0 0 0.5 0.5 1 1 1 1
  spline S136 degree 3 poles (-12.6586, -95.8836) (-12.3667, -95.9221) (-12.0746, -95.9593) (-11.4902, -96.0311) (-11.1978, -96.0656) (-10.9053, -96.0988) knots 0 0 0 0 0.5 0.5 1 1 1 1
  spline S137 degree 3 poles (-15.078, -100.086) (-14.6096, -99.4257) (-14.1727, -98.7437) (-13.3649, -97.3405) (-12.9944, -96.6202) (-12.6586, -95.8836) knots 0 0 0 0 0.5 0.5 1 1 1 1
  arc A47 (-16.9035, -99.7939) -> (-15.078, -100.086) centre (0, 0) ccw
  spline S138 degree 3 poles (-17.8909, -95.0464) (-17.8017, -95.851) (-17.6745, -96.651) (-17.3448, -98.2361) (-17.1425, -99.0205) (-16.9035, -99.7939) knots 0 0 0 0 0.5 0.5 1 1 1 1
  spline S139 degree 3 poles (-19.6239, -94.7038) (-19.3356, -94.7635) (-19.047, -94.8219) (-18.4694, -94.9361) (-18.1803, -94.9919) (-17.8909, -95.0464) knots 0 0 0 0 0.5 0.5 1 1 1 1
  spline S140 degree 3 poles (-22.3436, -98.7184) (-21.8283, -98.0941) (-21.3428, -97.4457) (-20.4346, -96.1052) (-20.0126, -95.4139) (-19.6239, -94.7038) knots 0 0 0 0 0.5 0.5 1 1 1 1
  arc A48 (-24.1429, -98.2938) -> (-22.3436, -98.7184) centre (0, 0) ccw
  spline S141 degree 3 poles (-24.7811, -93.4869) (-24.7509, -94.2959) (-24.6824, -95.103) (-24.4693, -96.708) (-24.3248, -97.505) (-24.1429, -98.2938) knots 0 0 0 0 0.5 0.5 1 1 1 1
  spline S142 degree 3 poles (-26.4845, -93.0187) (-26.2013, -93.0993) (-25.9178, -93.1786) (-25.35, -93.3347) (-25.0657, -93.4114) (-24.7811, -93.4869) knots 0 0 0 0 0.5 0.5 1 1 1 1
  spline S143 degree 3 poles (-29.49, -96.824) (-28.9304, -96.239) (-28.3989, -95.6278) (-27.3954, -94.3572) (-26.9239, -93.6986) (-26.4845, -93.0187) knots 0 0 0 0 0.5 0.5 1 1 1 1
  arc A49 (-31.2535, -96.2693) -> (-29.49, -96.824) centre (0, 0) ccw
  spline S144 degree 3 poles (-31.5391, -91.4286) (-31.568, -92.2376) (-31.5586, -93.0476) (-31.4632, -94.6638) (-31.3773, -95.4693) (-31.2535, -96.2693) knots 0 0 0 0 0.5 0.5 1 1 1 1
  spline S145 degree 3 poles (-33.2037, -90.8373) (-32.9272, -90.9384) (-32.6502, -91.0382) (-32.0953, -91.2353) (-31.8175, -91.3326) (-31.5391, -91.4286) knots 0 0 0 0 0.5 0.5 1 1 1 1
  spline S146 degree 3 poles (-36.479, -94.4131) (-35.8783, -93.8705) (-35.3035, -93.2997) (-34.2099, -92.1058) (-33.6917, -91.4833) (-33.2037, -90.8373) knots 0 0 0 0 0.5 0.5 1 1 1 1
  arc A50 (-38.1973, -93.7311) -> (-36.479, -94.4131) centre (0, 0) ccw
  spline S147 degree 3 poles (-38.1289, -88.8825) (-38.2167, -89.6872) (-38.2664, -90.4957) (-38.2893, -92.1146) (-38.2624, -92.9242) (-38.1973, -93.7311) knots 0 0 0 0 0.5 0.5 1 1 1 1
  spline S148 degree 3 poles (-39.7459, -88.1713) (-39.4774, -88.2922) (-39.2085, -88.412) (-38.6695, -88.6491) (-38.3994, -88.7664) (-38.1289, -88.8825) knots 0 0 0 0 0.5 0.5 1 1 1 1
  spline S149 degree 3 poles (-43.2734, -91.4984) (-42.6347, -91.0011) (-42.0198, -90.4738) (-40.8419, -89.3629) (-40.2796, -88.7799) (-39.7459, -88.1713) knots 0 0 0 0 0.5 0.5 1 1 1 1
  arc A51 (-44.9373, -90.6928) -> (-43.2734, -91.4984) centre (0, 0) ccw
  spline S150 degree 3 poles (-44.5151, -85.8621) (-44.6615, -86.6583) (-44.7701, -87.461) (-44.9111, -89.074) (-44.9434, -89.8833) (-44.9373, -90.6928) knots 0 0 0 0 0.5 0.5 1 1 1 1
  spline S151 degree 3 poles (-46.0759, -85.0348) (-45.817, -85.175) (-45.5575, -85.3141) (-45.0373, -85.5899) (-44.7765, -85.7266) (-44.5151, -85.8621) knots 0 0 0 0 0.5 0.5 1 1 1 1
  spline S152 degree 3 poles (-49.8369, -88.0956) (-49.1636, -87.6462) (-48.5119, -87.1652) (-47.2561, -86.1432) (-46.6527, -85.6028) (-46.0759, -85.0348) knots 0 0 0 0 0.5 0.5 1 1 1 1
  arc A52 (-51.4376, -87.1707) -> (-49.8369, -88.0956) centre (0, 0) ccw
  spline S153 degree 3 poles (-50.6639, -82.3837) (-50.868, -83.1671) (-51.0349, -83.9597) (-51.2933, -85.558) (-51.3845, -86.3629) (-51.4376, -87.1707) knots 0 0 0 0 0.5 0.5 1 1 1 1
  spline S154 degree 3 poles (-52.1601, -81.4446) (-51.9122, -81.6034) (-51.6635, -81.761) (-51.1648, -82.0741) (-50.9147, -82.2294) (-50.6639, -82.3837) knots 0 0 0 0 0.5 0.5 1 1 1 1
  spline S155 degree 3 poles (-56.1346, -84.2227) (-55.4302, -83.8237) (-54.7451, -83.3916) (-53.4181, -82.464) (-52.7769, -81.969) (-52.1601, -81.4446) knots 0 0 0 0 0.5 0.5 1 1 1 1
  arc A53 (-57.6634, -83.1834) -> (-56.1346, -84.2227) centre (0, 0) ccw
  spline S156 degree 3 poles (-56.5424, -78.4657) (-56.8031, -79.2321) (-57.0275, -80.0104) (-57.4018, -81.5856) (-57.5515, -82.3817) (-57.6634, -83.1834) knots 0 0 0 0 0.5 0.5 1 1 1 1
  spline S157 degree 3 poles (-57.9661, -77.4199) (-57.7304, -77.5963) (-57.4939, -77.7717) (-57.0193, -78.1203) (-56.7813, -78.2935) (-56.5424, -78.4657) knots 0 0 0 0 0.5 0.5 1 1 1 1
  spline S158 degree 3 poles (-62.1327, -79.9005) (-61.401, -79.5539) (-60.6862, -79.173) (-59.295, -78.3447) (-58.6194, -77.8979) (-57.9661, -77.4199) knots 0 0 0 0 0.5 0.5 1 1 1 1
  arc A54 (-63.5816, -78.7524) -> (-62.1327, -79.9005) centre (0, 0) ccw
  spline S159 degree 3 poles (-62.1192, -74.129) (-62.4352, -74.8743) (-62.7157, -75.6342) (-63.204, -77.1779) (-63.4115, -77.9609) (-63.5816, -78.7524) knots 0 0 0 0 0.5 0.5 1 1 1 1
  spline S160 degree 3 poles (-63.4627, -72.9821) (-63.2405, -73.1753) (-63.0175, -73.3675) (-62.5696, -73.7498) (-62.3448, -73.9399) (-62.1192, -74.129) knots 0 0 0 0 0.5 0.5 1 1 1 1
  spline S161 degree 3 poles (-67.7993, -75.1519) (-67.0443, -74.8597) (-66.3036, -74.5319) (-64.8556, -73.8074) (-64.1492, -73.4111) (-63.4627, -72.9821) knots 0 0 0 0 0.5 0.5 1 1 1 1
  arc A55 (-69.1606, -73.9011) -> (-67.7993, -75.1519) centre (0, 0) ccw
  spline S162 degree 3 poles (-67.3645, -69.3969) (-67.7341, -70.1171) (-68.0693, -70.8545) (-68.669, -72.3584) (-68.9331, -73.1242) (-69.1606, -73.9011) knots 0 0 0 0 0.5 0.5 1 1 1 1
  spline S163 degree 3 poles (-68.6208, -68.1549) (-68.4133, -68.3638) (-68.2049, -68.5718) (-67.7861, -68.9857) (-67.5758, -69.1918) (-67.3645, -69.3969) knots 0 0 0 0 0.5 0.5 1 1 1 1
  spline S164 degree 3 poles (-73.1041, -70.0024) (-72.3299, -69.7661) (-71.5672, -69.4933) (-70.0702, -68.8764) (-69.3368, -68.5327) (-68.6208, -68.1549) knots 0 0 0 0 0.5 0.5 1 1 1 1
  arc A56 (-74.3705, -68.6556) -> (-73.1041, -70.0024) centre (0, 0) ccw
  spline S165 degree 3 poles (-72.2505, -64.2944) (-72.6716, -64.9858) (-73.0598, -65.6967) (-73.7677, -67.1529) (-74.0869, -67.8973) (-74.3705, -68.6556) knots 0 0 0 0 0.5 0.5 1 1 1 1
  spline S166 degree 3 poles (-73.4127, -62.9641) (-73.221, -63.1876) (-73.0283, -63.4102) (-72.6409, -63.8536) (-72.4462, -64.0745) (-72.2505, -64.2944) knots 0 0 0 0 0.5 0.5 1 1 1 1
  spline S167 degree 3 poles (-78.019, -64.4794) (-77.2295, -64.3002) (-76.449, -64.0838) (-74.911, -63.5778) (-74.1544, -63.2886) (-73.4127, -62.9641) knots 0 0 0 0 0.5 0.5 1 1 1 1
  arc A57 (-79.1836, -63.0437) -> (-78.019, -64.4794) centre (0, 0) ccw
  spline S168 degree 3 poles (-76.7509, -58.849) (-77.2214, -59.5078) (-77.6604, -60.1884) (-78.4727, -61.589) (-78.8455, -62.3082) (-79.1836, -63.0437) knots 0 0 0 0 0.5 0.5 1 1 1 1
  spline S169 degree 3 poles (-77.8129, -57.4374) (-77.6381, -57.6742) (-77.4622, -57.9103) (-77.1081, -58.3809) (-76.9301, -58.6153) (-76.7509, -58.849) knots 0 0 0 0 0.5 0.5 1 1 1 1
  spline S170 degree 3 poles (-82.5175, -58.6124) (-81.7171, -58.4913) (-80.9228, -58.3324) (-79.352, -57.9401) (-78.5763, -57.7069) (-77.8129, -57.4374) knots 0 0 0 0 0.5 0.5 1 1 1 1
  arc A58 (-83.5743, -57.0955) -> (-82.5175, -58.6124) centre (0, 0) ccw
  spline S171 degree 3 poles (-80.8419, -53.0895) (-81.3592, -53.7122) (-81.8467, -54.359) (-82.7591, -55.6966) (-83.1833, -56.3866) (-83.5743, -57.0955) knots 0 0 0 0 0.5 0.5 1 1 1 1
  spline S172 degree 3 poles (-81.798, -51.6042) (-81.6409, -51.8532) (-81.4827, -52.1015) (-81.164, -52.5966) (-81.0035, -52.8434) (-80.8419, -53.0895) knots 0 0 0 0 0.5 0.5 1 1 1 1
  spline S173 degree 3 poles (-86.5758, -52.4326) (-85.7687, -52.3703) (-84.9649, -52.2698) (-83.3697, -51.9932) (-82.579, -51.8172) (-81.798, -51.6042) knots 0 0 0 0 0.5 0.5 1 1 1 1
  arc A59 (-87.519, -50.8427) -> (-86.5758, -52.4326) centre (0, 0) ccw
  spline S174 degree 3 poles (-84.5015, -47.0468) (-85.0629, -47.6301) (-85.5964, -48.2396) (-86.6039, -49.507) (-87.0774, -50.1642) (-87.519, -50.8427) knots 0 0 0 0 0.5 0.5 1 1 1 1
  spline S175 degree 3 poles (-85.3467, -45.4956) (-85.2082, -45.7554) (-85.0685, -46.0146) (-84.7867, -46.5317) (-84.6447, -46.7896) (-84.5015, -47.0468) knots 0 0 0 0 0.5 0.5 1 1 1 1
  spline S176 degree 3 poles (-90.1722, -45.9731) (-89.3627, -45.9699) (-88.5537, -45.9283) (-86.9425, -45.7689) (-86.1411, -45.6511) (-85.3467, -45.4956) knots 0 0 0 0 0.5 0.5 1 1 1 1
  arc A60 (-90.9968, -44.3185) -> (-90.1722, -45.9731) centre (0, 0) ccw
  spline S177 degree 3 poles (-87.7103, -40.7531) (-88.3127, -41.2938) (-88.8893, -41.8628) (-89.9866, -43.0532) (-90.5068, -43.6741) (-90.9968, -44.3185) knots 0 0 0 0 0.5 0.5 1 1 1 1
  spline S178 degree 3 poles (-88.4399, -39.1443) (-88.3208, -39.4136) (-88.2004, -39.6823) (-87.9572, -40.2185) (-87.8343, -40.4861) (-87.7103, -40.7531) knots 0 0 0 0 0.5 0.5 1 1 1 1
  spline S179 degree 3 poles (-93.2875, -39.2683) (-92.4799, -39.3242) (-91.6701, -39.3418) (-90.0515, -39.3004) (-89.2436, -39.2414) (-88.4399, -39.1443) knots 0 0 0 0 0.5 0.5 1 1 1 1
  arc A61 (-93.9891, -37.558) -> (-93.2875, -39.2683) centre (0, 0) ccw
  spline S180 degree 3 poles (-90.4511, -34.2419) (-91.0914, -34.7372) (-91.7079, -35.2626) (-92.8893, -36.3698) (-93.4534, -36.951) (-93.9891, -37.558) knots 0 0 0 0 0.5 0.5 1 1 1 1
  spline S181 degree 3 poles (-91.0614, -32.5842) (-90.9622, -32.8614) (-90.8617, -33.1382) (-90.6583, -33.6908) (-90.5553, -33.9666) (-90.4511, -34.2419) knots 0 0 0 0 0.5 0.5 1 1 1 1
  spline S182 degree 3 poles (-95.905, -32.354) (-95.1036, -32.4687) (-94.2973, -32.5454) (-92.68, -32.6222) (-91.87, -32.6224) (-91.0614, -32.5842) knots 0 0 0 0 0.5 0.5 1 1 1 1
  arc A62 (-96.4799, -30.597) -> (-95.905, -32.354) centre (0, 0) ccw
  spline S183 degree 3 poles (-92.7093, -27.5481) (-93.384, -27.9953) (-94.0373, -28.4743) (-95.2963, -29.4923) (-95.9013, -30.0308) (-96.4799, -30.597) knots 0 0 0 0 0.5 0.5 1 1 1 1
  spline S184 degree 3 poles (-93.1969, -25.8502) (-93.1182, -26.1339) (-93.0383, -26.4173) (-92.8757, -26.9833) (-92.7931, -27.2659) (-92.7093, -27.5481) knots 0 0 0 0 0.5 0.5 1 1 1 1
  spline S185 degree 3 poles (-98.0109, -25.2671) (-97.22, -25.44) (-96.4214, -25.5753) (-94.814, -25.77) (-94.0062, -25.8293) (-93.1969, -25.8502) knots 0 0 0 0 0.5 0.5 1 1 1 1
  arc A63 (-98.456, -23.4728) -> (-98.0109, -25.2671) centre (0, 0) ccw
  spline S186 degree 3 poles (-94.4728, -20.7072) (-95.1784, -21.104) (-95.8649, -21.534) (-97.1949, -22.4574) (-97.8376, -22.9503) (-98.456, -23.4728) knots 0 0 0 0 0.5 0.5 1 1 1 1
  spline S187 degree 3 poles (-94.8353, -18.9783) (-94.7775, -19.267) (-94.7184, -19.5555) (-94.5976, -20.1318) (-94.5359, -20.4197) (-94.4728, -20.7072) knots 0 0 0 0 0.5 0.5 1 1 1 1
  spline S188 degree 3 poles (-99.5938, -18.0454) (-98.8176, -18.2755) (-98.031, -18.4687) (-96.4422, -18.7803) (-95.6408, -18.8983) (-94.8353, -18.9783) knots 0 0 0 0 0.5 0.5 1 1 1 1
  arc A64 (-99.9067, -16.2234) -> (-99.5938, -18.0454) centre (0, 0) ccw
  spline S189 degree 3 poles (-95.7323, -13.7559) (-96.465, -14.1002) (-97.181, -14.4789) (-98.5749, -15.3027) (-99.2519, -15.7474) (-99.9067, -16.2234) knots 0 0 0 0 0.5 0.5 1 1 1 1
  spline S190 degree 3 poles (-95.9676, -12.0052) (-95.931, -12.2973) (-95.8932, -12.5893) (-95.8147, -13.1729) (-95.7742, -13.4645) (-95.7323, -13.7559) knots 0 0 0 0 0.5 0.5 1 1 1 1
  spline S191 degree 3 poles (-100.6453, -10.7273) (-99.888, -11.0135) (-99.1176, -11.2637) (-97.5558, -11.6903) (-96.7652, -11.8666) (-95.9676, -12.0052) knots 0 0 0 0 0.5 0.5 1 1 1 1
  arc A65 (-100.8245, -8.8874) -> (-100.6453, -10.7273) centre (0, 0) ccw
  spline S192 degree 3 poles (-96.4811, -6.7312) (-97.2369, -7.0211) (-97.9787, -7.3465) (-99.4289, -8.0664) (-100.1366, -8.4605) (-100.8245, -8.8874) knots 0 0 0 0 0.5 0.5 1 1 1 1
  spline S193 degree 3 poles (-96.5879, -4.968) (-96.5728, -5.262) (-96.5563, -5.556) (-96.5207, -6.1437) (-96.5015, -6.4375) (-96.4811, -6.7312) knots 0 0 0 0 0.5 0.5 1 1 1 1
  spline S194 degree 3 poles (-101.1599, -3.3521) (-100.4255, -3.6928) (-99.6754, -3.9985) (-98.1489, -4.538) (-97.3732, -4.7715) (-96.5879, -4.968) knots 0 0 0 0 0.5 0.5 1 1 1 1
  arc A66 (-101.2042, -1.5039) -> (-101.1599, -3.3521) centre (0, 0) ccw
  spline S195 degree 3 poles (-96.715, 0.3294) (-97.49, 0.0955) (-98.2536, -0.1749) (-99.7525, -0.7871) (-100.487, -1.1284) (-101.2042, -1.5039) knots 0 0 0 0 0.5 0.5 1 1 1 1
  spline S196 degree 3 poles (-96.6929, 2.0957) (-96.6992, 1.8014) (-96.7043, 1.507) (-96.7117, 0.9182) (-96.714, 0.6238) (-96.715, 0.3294) knots 0 0 0 0 0.5 0.5 1 1 1 1
  spline S197 degree 3 poles (-101.1347, 4.0411) (-100.4271, 3.6477) (-99.7014, 3.288) (-98.2183, 2.6385) (-97.4618, 2.349) (-96.6929, 2.0957) knots 0 0 0 0 0.5 0.5 1 1 1 1
  arc A67 (-101.044, 5.8875) -> (-101.1347, 4.0411) centre (0, 0) ccw
  spline S198 degree 3 poles (-96.433, 7.3883) (-97.223, 7.2116) (-98.0042, 6.9976) (-99.5438, 6.4965) (-100.3013, 6.2097) (-101.044, 5.8875) knots 0 0 0 0 0.5 0.5 1 1 1 1
  spline S199 degree 3 poles (-96.2819, 9.1483) (-96.3098, 8.8552) (-96.3363, 8.562) (-96.3866, 7.9753) (-96.4105, 7.6818) (-96.433, 7.3883) knots 0 0 0 0 0.5 0.5 1 1 1 1
  spline S200 degree 3 poles (-100.5699, 11.4126) (-99.893, 10.9687) (-99.1954, 10.557) (-97.7637, 9.8009) (-97.0303, 9.457) (-96.2819, 9.1483) knots 0 0 0 0 0.5 0.5 1 1 1 1
  arc A68 (-100.3447, 13.2475) -> (-100.5699, 11.4126) centre (0, 0) ccw
  spline S201 degree 3 poles (-95.6364, 14.4077) (-96.4372, 14.2892) (-97.232, 14.1328) (-98.804, 13.7454) (-99.5805, 13.5146) (-100.3447, 13.2475) knots 0 0 0 0 0.5 0.5 1 1 1 1
  spline S202 degree 3 poles (-95.3573, 16.152) (-95.4065, 15.8617) (-95.4543, 15.5712) (-95.5474, 14.9898) (-95.5925, 14.6988) (-95.6364, 14.4077) knots 0 0 0 0 0.5 0.5 1 1 1 1
  spline S203 degree 3 poles (-99.4685, 18.7233) (-98.8258, 18.2311) (-98.1602, 17.7696) (-96.7874, 16.9111) (-96.0812, 16.5145) (-95.3573, 16.152) knots 0 0 0 0 0.5 0.5 1 1 1 1
  arc A69 (-99.11, 20.5369) -> (-99.4685, 18.7233) centre (0, 0) ccw
  spline S204 degree 3 poles (-94.3296, 21.3503) (-95.1369, 21.2905) (-95.941, 21.1926) (-97.5371, 20.921) (-98.3283, 20.7475) (-99.11, 20.5369) knots 0 0 0 0 0.5 0.5 1 1 1 1
  spline S205 degree 3 poles (-93.9239, 23.0696) (-93.9941, 22.7836) (-94.063, 22.4974) (-94.1983, 21.9243) (-94.2646, 21.6374) (-94.3296, 21.3503) knots 0 0 0 0 0.5 0.5 1 1 1 1
  spline S206 degree 3 poles (-97.8365, 25.9341) (-97.2314, 25.3963) (-96.6012, 24.8874) (-95.2948, 23.931) (-94.6194, 23.4839) (-93.9239, 23.0696) knots 0 0 0 0 0.5 0.5 1 1 1 1
  arc A70 (-97.3465, 27.7167) -> (-97.8365, 25.9341) centre (0, 0) ccw
  spline S207 degree 3 poles (-92.5195, 28.1789) (-93.329, 28.1783) (-94.1381, 28.1393) (-95.7498, 27.9849) (-96.5515, 27.8697) (-97.3465, 27.7167) knots 0 0 0 0 0.5 0.5 1 1 1 1